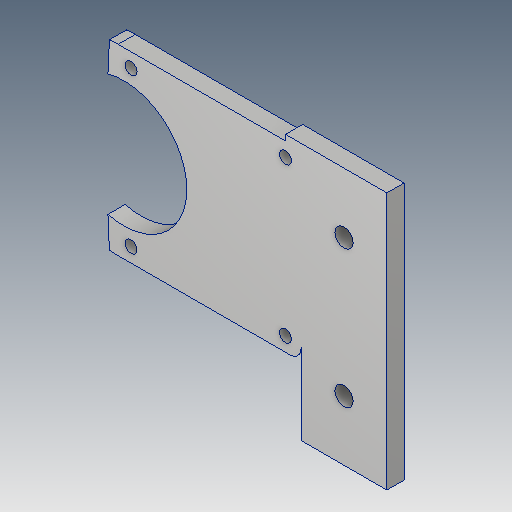
# Autodesk Inventor part: デュアルサーボつなぎフレーム_アルミ(A2017)_t1.5
Saved by Autodesk Inventor 2019.4 (Build 234330000, 330)
## iProperties
Created: 2019-06-16
Part Number: デュアルサーボつなぎフレーム_アルミ(A2017)_t1.5
Material: アルミニウム 6061
Document SubType Name: Modeling
Designer: 長谷川翔一
Density: 2.7 g/cm^3
Appearance: アルミニウム - フラット
Mass: 12.0813 g
Surface Area: 37.8901 cm^2
Volume: 4.47456 cm^3
Author: 長谷川翔一
Autodesk Inventor part; units mm, degrees
ref_plane "YZ Plane" through (0, 0, 0) normal (1, 0, 0) x (0, 1, 0)
ref_plane "XZ Plane" through (0, 0, 0) normal (0, 1, 0) x (-1, 0, 0)
ref_plane "XY Plane" through (0, 0, 0) normal (0, 0, 1) x (1, 0, 0)
sketch "スケッチ1" plane through (0, 0, 0) normal (0, 0, 1) x (1, 0, 0)
  circle A0 centre (-18.2979, -11.3675) radius 1.05 construction
  circle A1 centre (-0.7979, 13.5) radius 1.05 construction
  circle A2 centre (12.2021, -13.5) radius 1.05 construction
  circle A3 centre (-18.2979, 10.6325) radius 1.05 construction
  circle A4 centre (-10.7975, 0) radius 1.3 construction
  circle A5 centre (-9.5382, 13.5) radius 1.05 projected
  circle A6 centre (-9.5382, -13.5) radius 1.05 projected
  circle A7 centre (17.4618, 13.5) radius 1.05 projected
  circle A8 centre (17.4618, -13.5) radius 1.05 projected
  line L0 (-11.7979, -16) -> (18.2021, -16) projected
  arc A9 (18.2021, -16) -> (20.2021, -14) centre (18.2021, -14) ccw projected
  line L1 (20.2021, -14) -> (20.2021, 14) projected
  arc A10 (20.2021, 14) -> (18.2021, 16) centre (18.2021, 14) ccw projected
  line L2 (18.2021, 16) -> (-11.7979, 16) projected
  line L3 (-22.7979, 0) -> (0, 0) construction
  line L4 (0, 0) -> (13.5202, -23.4176) construction
  line L5 (-22.7979, 0) -> (-32.6431, 0) construction
  line L6 (9.2376, -16) -> (3.5384, -19.2904) construction
  line L7 (11.7376, -20.3301) -> (14.3357, -18.8301) construction
  line L8 (9.2376, 16) -> (3.5384, 19.2904) construction
  line L9 (11.7376, 20.3301) -> (14.3357, 18.8301) construction
  circle A11 centre (17.4618, -13.5) radius 2.5 construction
  circle A12 centre (17.4618, 13.5) radius 2.5 construction
  line L10 (3.6668, -16) -> (18.2021, -16)
  arc A13 (18.2021, -16) -> (20.2021, -14) centre (18.2021, -14) ccw
  line L11 (3.6668, 16) -> (18.2021, 16)
  arc A14 (20.2021, 14) -> (18.2021, 16) centre (18.2021, 14) ccw
  line L12 (-5.7966, 16) -> (-11.7979, 16)
  arc A15 (-11.7979, 16) -> (-13.3279, 15.9267) centre (-11.7979, 0) ccw
  line L13 (-5.7966, -16) -> (-11.7979, -16)
  arc A16 (-13.3279, -15.9267) -> (-11.7979, -16) centre (-11.7979, 0) ccw
  arc A17 (-13.5809, -10.642) -> (-13.5809, 10.642) centre (-10.7975, 0) ccw
  line L14 (-13.3279, -15.9267) -> (-13.5809, -10.642)
  line L15 (-13.5809, 10.642) -> (-13.3279, 15.9267)
  line L16 (20.2021, 0) -> (35.2021, 0) construction
  line L17 (20.2021, -22.5) -> (20.2021, -17.0694)
  line L18 (20.2021, -9.9306) -> (20.2021, 9.9306)
  line L19 (20.2021, 0) -> (35.2021, 0)
  line L20 (20.2021, -17.0694) -> (20.2021, -14)
  line L21 (17.4618, 17) -> (35.2021, 17)
  line L22 (20.2021, 14) -> (20.2021, -28)
  line L23 (20.2021, 17) -> (65.2021, 17) construction
  line L24 (20.2021, -28) -> (35.2021, -28)
  line L25 (35.2021, -28) -> (35.2021, 17)
  line L26 (27.7021, -28) -> (27.7021, 17) construction
  line L27 (27.7021, -5.5) -> (20.2021, -5.5) construction
  circle A18 centre (27.7021, -17.5) radius 1.6
  circle A19 centre (27.7021, 6.5) radius 1.6
  line L28 (17.4618, 13.5) -> (17.4618, 14.55)
  line L29 (17.4618, 16) -> (17.4618, 17)
  point P0 (-22.7979, -6.4363)
  point P1 (15.7302, -16)
  point P2 (13.5202, 23.4176)
  point P3 (15.7302, 16)
  dimension "d0" = 120
  dimension "d7" = 5
  dimension "d10" = 5
  dimension "d24" = 22
  dimension "d28" = 15
  dimension "d38" = 3.5
  dimension "d39" = 45
  dimension "d40" = 90
  dimension "d41" = 15
  dimension "d42" = 2.7403
  dimension "d43" = 3.2
  dimension "d44" = 12
  constraints: 54 end point, 13 point on line, 12 point on circle, 9 centre point, 8 symmetric about line, 6 tangent, 4 horizontal, 4 perpendicular, 4 vertical, 3 coincident, 3 midpoint, 2 collinear, 1 concentric, 1 vertical alignment, 2 other
  measures "d0" angle of L4 L3
  measures "d7" diameter of A11
  measures "d10" diameter of A12
  measures "d24" diameter of A17
  measures "d28" distance of L16.start L16.end
  measures "d38" distance of L28.start L21.start
  measures "d39" distance of L23.start L22.end
  measures "d40" angle of L22 L23
  measures "d41" distance of L22.end L24.end
  measures "d42" distance from line of point (17.462, 13.5) L22
  measures "d43" diameter of A18
  measures "d44" distance from line of L27 A18.centre
extrude "押し出し5" add sketch "スケッチ1" along normal blind 3
